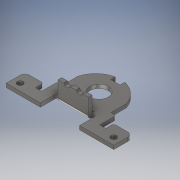
# Autodesk Inventor part: Część3
Saved by Autodesk Inventor 2017 SP1 (Build 210196100, 196)
## iProperties
Created: 2021-01-31
Part Number: Część3
Material: Stal
Document SubType Name: Modeling
Designer: Napoleon
Mass: 7.57161 g
Surface Area: 15.6917 cm^2
Volume: 0.964537 cm^3
Density: 7.85 g/cm^3
Appearance: Galwanizowana
Author: Napoleon
Autodesk Inventor part; units mm, degrees
ref_plane "YZ Plane" through (0, 0, 0) normal (1, 0, 0) x (0, 1, 0)
ref_plane "XZ Plane" through (0, 0, 0) normal (0, 1, 0) x (-1, 0, 0)
ref_plane "XY Plane" through (0, 0, 0) normal (0, 0, 1) x (1, 0, 0)
sketch "Szkic1" plane through (0, 0, 0) normal (0, 0, 1) x (1, 0, 0)
  circle A0 centre (0, 0) radius 4
  line L0 (-2, 7.05) -> (2, 7.05)
  line L1 (-2, 7.05) -> (-2, 9.05)
  line L2 (2, 7.05) -> (2, 9.05)
  line L3 (-6.525, -11.1) -> (6.525, -11.1)
  line L4 (10.3, 1.325) -> (10.3, -5.175)
  line L5 (12.525, -5.175) -> (12.525, -12.175)
  line L6 (12.525, -12.175) -> (15.125, -12.175)
  line L7 (15.125, -12.175) -> (15.125, -8.775)
  line L8 (15.125, -8.775) -> (23.125, -8.775)
  line L9 (6.525, -11.1) -> (6.525, -9.5)
  line L10 (6.525, -9.5) -> (8.425, -9.5)
  line L11 (-6.525, -9.5) -> (-8.425, -9.5)
  line L12 (-6.525, -9.5) -> (-6.525, -11.1)
  line L13 (12.525, -5.175) -> (10.3, -5.175)
  line L14 (23.125, -16.775) -> (8.425, -16.775)
  arc A1 (10.3, 1.325) -> (2, 9.05) centre (-0.2722, -1.7128) ccw
  line L15 (8.425, -16.775) -> (8.425, -9.5)
  line L16 (23.125, -16.775) -> (23.125, -8.775)
  line L17 (-10.3, 1.325) -> (-10.3, -5.175)
  line L18 (-12.525, -5.175) -> (-12.525, -12.175)
  line L19 (-12.525, -12.175) -> (-15.125, -12.175)
  line L20 (-15.125, -12.175) -> (-15.125, -8.775)
  line L21 (-15.125, -8.775) -> (-23.125, -8.775)
  line L22 (-12.525, -5.175) -> (-10.3, -5.175)
  line L23 (-23.125, -16.775) -> (-8.425, -16.775)
  arc A2 (-2, 9.05) -> (-10.3, 1.325) centre (0.2722, -1.7128) ccw
  line L24 (-8.425, -16.775) -> (-8.425, -9.5)
  line L25 (-23.125, -16.775) -> (-23.125, -8.775)
  dimension "d2" = 4
  dimension "d4" = 2
  dimension "d8" = 6.5
  dimension "d11" = 7
  dimension "d12" = 2.6
  dimension "d13" = 3.4
  dimension "d14" = 8
  dimension "d17" = 1.6
  dimension "d66" = 11
  constraints: 52 end point, 7 vertical, 5 perpendicular, 4 point on circle, 3 centre point, 2 horizontal
  measures "d2" distance of L0.start L0.end
  measures "d4" distance of L0.start L1.end
  measures "d8" distance of L4.start L4.end
  measures "d11" distance of L5.start L5.end
  measures "d12" distance of L5.end L6.end
  measures "d13" distance of L6.end L7.end
  measures "d14" distance of L7.end L8.end
  measures "d17" distance of L3.end L9.end
  measures "d66" radius of A1
extrude "Wyciągnięcie proste1" add sketch "Szkic1" along normal mid plane 1.6
fillet "Zaokrąglenie1" radius 2 2 edges at (23.125, -8.775, 0) (-23.125, -8.775, 0)
fillet "Zaokrąglenie2" radius 1 4 edges at (12.525, -5.175, 0) (15.125, -8.775, 0) (-15.125, -8.775, 0) (-12.525, -5.175, 0)
fillet "Zaokrąglenie3" radius 1 2 edges at (-8.425, -9.5, 0) (8.425, -9.5, 0)
sketch "Szkic2" plane through (0, 0, 0.8) normal (0, 0, 1) x (1, 0, 0)
  line L0 (-6.525, -9.5) -> (-6.525, -11.1)
  line L1 (-6.525, -11.1) -> (6.525, -11.1)
  line L2 (6.525, -11.1) -> (6.525, -9.5)
  line L3 (6.525, -9.5) -> (-6.525, -9.5)
  constraints: 8 end point, 1 horizontal
extrude "Wyciągnięcie proste2" add sketch "Szkic2" along normal blind 6.75
fillet "Zaokrąglenie4" radius 1.6 1 edges at (0, -11.1, -0.8) curvature continuous yes
sketch "Szkic3" plane through (0, 0, 0.8) normal (0, 0, 1) x (1, 0, 0)
  line L0 (-6.525, -9.5) -> (6.525, -9.5)
  line L1 (6.525, -9.5) -> (6.525, -8.5)
  line L2 (6.525, -8.5) -> (-6.525, -8.5)
  line L3 (-6.525, -9.5) -> (-6.525, -8.5)
  dimension "d44" = 1
  constraints: 8 end point, 2 perpendicular, 1 vertical
  measures "d44" distance of L0.end L1.end
extrude "Wyciągnięcie proste3" cut sketch "Szkic3" against normal blind 0.2
sketch "Szkic4" plane through (-6.525, -11.1, 7.55) normal (0, -1, 0) x (1, 0, 0)
  arc A0 (2.5, 0) -> (5.275, 0) centre (3.8875, 0.4626) ccw
  arc A1 (7.775, 0) -> (10.55, 0) centre (9.1625, 0.4626) ccw
  line L0 (2.5, 0) -> (5.275, 0)
  line L1 (7.775, 0) -> (10.55, 0)
  constraints: 4 end point, 4 point on circle, 2 centre point
extrude "Wyciągnięcie proste4" cut sketch "Szkic4" against normal through all
fillet "Zaokrąglenie5" radius 0.1 4 edges at (4.025, -10.3, 7.55) (-4.025, -10.3, 7.55) (-1.25, -10.3, 7.55) (1.25, -10.3, 7.55)
hole "Otwór4" at (-20.125, -13.775, 0.8) direction (0, 0, -1) diameter 2.459 end through all thread size "M3x0.5" class "6H" standard "ISO Metric profile"
hole "Otwór5" at (20.125, -13.775, 0.8) direction (0, 0, -1) diameter 2.459 end through all thread size "M3x0.5" class "6H" standard "ISO Metric profile"
